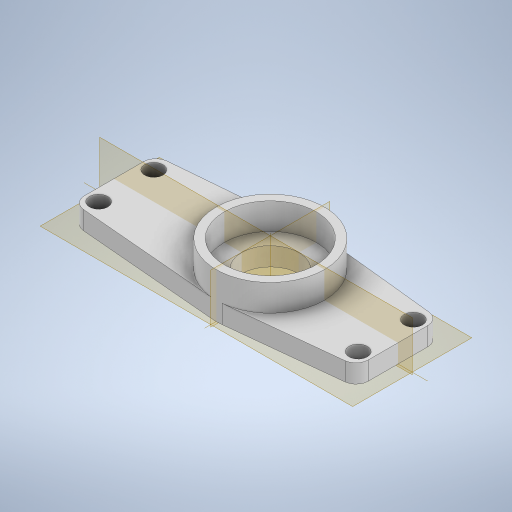
# Autodesk Inventor part: bearing_holder
Saved by Autodesk Inventor 2023 (Build 270158000, 158)
## iProperties
Created: 2022-06-30
Part Number: bearing_holder
Material: Generic
Document SubType Name: Modeling
Designer: Habib
Density: 1 g/cm^3
Appearance: Default
Author: Habib
Autodesk Inventor part; units mm, degrees
sketch "Sketch1" plane through (0, 0, 0) normal (0, 1, 0) x (-1, 0, 0)
  circle A0 centre (0, 0) radius 7
  line L0 (0, 0) -> (-31.25, 0)
  line L1 (-31.25, 0) -> (-31.25, -10)
  line L2 (-31.25, 0) -> (-31.25, 10)
  line L3 (-31.25, -10) -> (-1.4018, -13.1756)
  line L4 (-31.25, 10) -> (-1.4018, 13.1756)
  line L5 (0, 0) -> (38.25, 0)
  line L6 (38.25, 0) -> (38.25, -10)
  line L7 (38.25, -10) -> (1.1388, -13.1756)
  line L8 (38.25, 0) -> (38.25, 10)
  line L9 (38.25, 10) -> (1.4018, 13.1756)
  line L10 (-31.25, 0) -> (-28.25, 0)
  line L11 (-28.25, 0) -> (-28.25, -6.75)
  line L12 (-28.25, 0) -> (-28.25, 6.75)
  circle A1 centre (-28.25, -6.75) radius 2.25
  circle A2 centre (-28.25, 6.75) radius 2.25
  line L13 (38.25, 0) -> (35.25, 0)
  line L14 (35.25, 0) -> (35.25, -6.75)
  line L15 (35.25, 0) -> (35.25, 6.75)
  circle A3 centre (35.25, -6.75) radius 2.25
  circle A4 centre (35.25, 6.75) radius 2.25
  line L16 (1.1388, -13.1756) -> (-1.4018, -13.1756)
  line L17 (1.4018, 13.1756) -> (-1.4018, 13.1756)
  dimension "d2" = 14
  dimension "d3" = 31.25
  dimension "d4" = 10
  dimension "d5" = 10
  dimension "d6" = 38.25
  dimension "d7" = 10
  dimension "d8" = 10
  dimension "d9" = 3
  dimension "d10" = 6.75
  dimension "d11" = 6.75
  dimension "d12" = 4.5
  dimension "d13" = 4.5
  dimension "d14" = 3
  dimension "d15" = 6.75
  dimension "d16" = 6.75
  dimension "d17" = 4.5
  dimension "d18" = 4.5
  constraints: 36 end point, 5 centre point, 4 coincident, 3 horizontal, 3 perpendicular, 3 point on line, 3 vertical, 2 parallel
  measures "d2" diameter of A0
  measures "d3" distance of L0.start L0.end
  measures "d4" distance of L0.end L1.end
  measures "d5" distance of L0.end L2.end
  measures "d6" distance of L0.start L5.end
  measures "d7" distance of L5.end L6.end
  measures "d8" distance of L5.end L8.end
  measures "d9" distance of L0.end L10.end
  measures "d10" distance of L10.end L11.end
  measures "d11" distance of L10.end L12.end
  measures "d12" diameter of A1
  measures "d13" diameter of A2
  measures "d14" distance of L5.end L13.end
  measures "d15" distance of L13.end L14.end
  measures "d16" distance of L13.end L15.end
  measures "d17" diameter of A3
  measures "d18" diameter of A4
extrude "Extrusion1" add sketch "Sketch1" along normal blind 4.5 contours L5 L6 L7 L16 L3 L1 L0 A0 | A0 L0 L2 L4 L17 L9 L8 L5
sketch "Sketch2" plane through (0, 0, 0) normal (0, 1, 0) x (-1, 0, 0)
  circle A0 centre (0, 0) radius 13.25
  circle A1 centre (0, 0) radius 11.25
  dimension "d21" = 26.5
  dimension "d22" = 22.5
  constraints: 2 centre point, 2 coincident
  measures "d21" diameter of A0
  measures "d22" diameter of A1
extrude "Extrusion2" add sketch "Sketch2" along normal blind 11
fillet "Fillet1" radius 3 1 edges at (-38.25, 2.25, -10)
fillet "Fillet2" radius 3 3 edges at (-38.25, 2.25, 10) (31.25, 2.25, 10) (31.25, 2.25, -10)
body "Solid1"
